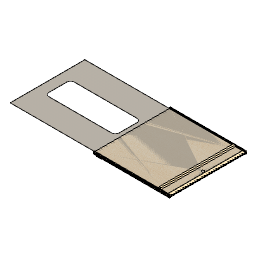
MKFG_DIYDoughLoader v2 (Autodesk Fusion 360 design; units mm, degrees)
Autodesk Fusion 360 part; units mm, degrees
sketch "Sketch1" plane through (0, 0, 0) normal (0, 1, 0) x (1, 0, 0) in component "ply_1/4_22x22"
  line L0 (-279.4, 279.4) -> (279.4, 279.4)
  line L1 (279.4, 279.4) -> (279.4, -279.4)
  line L2 (279.4, -279.4) -> (-279.4, -279.4)
  line L3 (-279.4, -279.4) -> (-279.4, 279.4)
  dimension "d1" = 558.8
  dimension "d2" = 558.8
  dimension "d3" = 279.4
  dimension "d4" = 279.4
  constraint horizontal L0
  constraint vertical L1
  constraint horizontal L2
  constraint vertical L3
  measures "d1" distance of L0.start L0.end
  measures "d2" distance of L0.start L2.end
  measures "d3" distance of origin L0
  measures "d4" distance of origin L3
extrude "Extrude1" add sketch "Sketch1" along normal blind 5.08 makes body 1 in component "ply_1/4_22x22"
sketch "Sketch1 (2)" plane through (0, 0, 0) normal (0, -1, 0) x (1, 0, 0) in component "Rails"
  line L0 (279.4, 279.4) -> (-279.4, 279.4)
  line L1 (-279.4, 279.4) -> (-279.4, -279.4)
  line L2 (-279.4, -279.4) -> (279.4, -279.4)
  line L3 (279.4, -279.4) -> (279.4, 279.4)
  line L4 (279.4, 273.05) -> (-279.4, 273.05)
  line L5 (-279.4, -273.05) -> (279.4, -273.05)
  dimension "d7" = -6.35
  dimension "d8" = -6.35
  constraint coincident L3 L5.end
  constraint perpendicular L3 L5
  constraint coincident L1 L5.start
  constraint coincident L3 L4.start
  constraint perpendicular L3 L4
  constraint coincident L1 L4.end
extrude "Extrude1'" add sketch "Sketch1 (2)" along normal blind 6.35 separate body contours L0 L1 L3 L4 | L1 L2 L3 L5 makes body 2 at (-93.1333, 0, -277.2833) makes body 3 at (-93.1333, 0, 275.1667) in component "Rails"
extrude "Extrude2" add sketch "Sketch1 (2)" against normal blind 6.35 from surface at -5.08 separate body contours L0 L1 L3 L4 | L1 L2 L3 L5 makes body 4 at (-93.1333, 5.08, -277.2833) makes body 5 at (-93.1333, 5.08, 275.1667) in component "Rails"
sketch "Sketch1 (3)" plane through (0, 0, -273.05) normal (0, 0, 1) x (1, 0, 0) in component "handle"
  line L0 (-279.4, 5.08) -> (279.4, 5.08)
  line L1 (279.4, 11.43) -> (-279.4, 11.43)
  line L2 (190.5, 5.08) -> (203.2, 5.08)
  line L3 (203.2, 5.08) -> (203.2, 17.78)
  line L4 (203.2, 17.78) -> (190.5, 17.78)
  line L5 (190.5, 17.78) -> (190.5, 5.08)
  line L6 (279.4, 5.08) -> (279.4, 11.43)
  line L7 (-279.4, 11.43) -> (-279.4, 5.08)
  dimension "d28" = 12.7
  dimension "d29" = 12.7
  dimension "d30" = 190.5
  constraint horizontal L2
  constraint vertical L3
  constraint horizontal L4
  constraint vertical L5
  constraint coincident L0 L2.start
  measures "d28" distance of L2.start L2.end
  measures "d29" distance of L2.start L4.end
  measures "d30" distance of origin L5
extrude "Extrude1''" add sketch "Sketch1 (3)" along normal blind 542.925 from surface at 1.5875 separate body contours L0 L1 L2 L3 L5 | L1 L3 L4 L5 makes body 6 in component "handle"
sketch "Sketch1 (4)" plane through (0, 5.08, 0) normal (0, 1, 0) x (-1, 0, 0) in component "Cloth"
  line L0 (279.4, 279.4) -> (-279.4, 279.4)
  line L1 (-279.4, -279.4) -> (279.4, -279.4)
  line L2 (-254, -271.4625) -> (279.4, -271.4625)
  line L3 (279.4, 271.4625) -> (-254, 271.4625)
  line L4 (-254, 271.4625) -> (-254, -271.4625)
  line L5 (279.4, -271.4625) -> (889, -271.4625)
  line L6 (304.8, -91.4625) -> (889, -91.4625)
  line L7 (889, -91.4625) -> (889, -271.4625)
  line L8 (889, -181.4625) -> (812.8, -181.4625) construction
  line L9 (889, -179.9625) -> (812.8, -179.9625)
  line L10 (889, -182.9625) -> (812.8, -182.9625)
  line L11 (812.8, -182.9625) -> (812.8, -179.9625)
  line L12 (279.4, 0) -> (325, 0) construction
  line L13 (304.8, 91.4625) -> (889, 91.4625)
  line L14 (279.4, 271.4625) -> (889, 271.4625)
  line L15 (889, 91.4625) -> (889, 271.4625)
  line L16 (889, 179.9625) -> (812.8, 179.9625)
  line L17 (889, 182.9625) -> (812.8, 182.9625)
  line L18 (812.8, 182.9625) -> (812.8, 179.9625)
  line L19 (889, -91.4625) -> (889, 91.4625)
  line L20 (812.8, -91.4625) -> (812.8, 91.4625)
  line L21 (-279.4, 279.4) -> (-279.4, -279.4)
  line L22 (279.4, -279.4) -> (279.4, 279.4)
  line L23 (304.8, -91.4625) -> (304.8, 91.4625)
  dimension "d43" = -7.9375
  dimension "d44" = -7.9375
  dimension "d47" = 609.6
  dimension "d48" = -180
  dimension "d49" = 76.2
  dimension "d50" = 1.5
  dimension "d51" = -1.5
  dimension "d56" = 76.2
  dimension "d59" = 25.4
  dimension "d60" = 25.4
  constraint coincident L3 L4.start
  constraint coincident L2 L4.end
  constraint perpendicular L2 L4
  constraint vertical L7
  constraint midpoint L7 L8.start
  constraint perpendicular L7 L8
  constraint perpendicular L9 L11
  constraint coincident L8.end L11
  constraint coincident L7 L10.start
  constraint coincident L7 L9.start
  constraint symmetric L2.end L12 L3.start
  constraint symmetric L5.end L12 L14.end
  constraint symmetric L6.start L12 L13.start
  constraint symmetric L6.end L12 L13.end
  constraint symmetric L9.start L12 L16.start
  constraint symmetric L9.end L12 L16.end
  constraint symmetric L10.start L12 L17.start
  constraint symmetric L10.end L12 L17.end
  constraint coincident L6 L20.start
  constraint coincident L13 L20.end
  constraint perpendicular L13 L20
  constraint midpoint L12.start L22
  constraint perpendicular L12 L22
  constraint coincident L2.end L22
  measures "d47" distance of L2.end L5.end
  measures "d49" distance of L8.start L8.end
  measures "d56" distance of L19 L20
  measures "d59" distance of L4 L21
  measures "d60" distance of L22 L23
extrude "Extrude1'''" add sketch "Sketch1 (4)" along normal blind 1.5 separate body contours L2 L3 L4 L22 | L5 L6 L7 L9 L10 L11 L13 L14 L15 L16 L17 L18 L22 L23 | L15 L16 L17 L18 | L7 L9 L10 L11 | L6 L13 L19 L20 makes body 7 in component "Cloth"
fillet "Fillet1" radius 25 4 edges at (-812.8, 5.83, -91.4625) (-812.8, 5.83, 91.4625) (-304.8, 5.83, -91.4625) (-304.8, 5.83, 91.4625) on bodies 7 in component "Cloth"
sketch "Sketch1 (5)" plane through (0, 0, 0) normal (0, -1, 0) x (1, 0, 0) in component "Bumpers_1/8x1/2"
  line L0 (279.4, 279.4) -> (-279.4, 279.4)
  line L1 (-279.4, 279.4) -> (-279.4, -279.4)
  line L2 (-279.4, -279.4) -> (279.4, -279.4)
  line L3 (279.4, -279.4) -> (279.4, 279.4)
  line L4 (-266.7, 279.4) -> (-266.7, -279.4)
  line L5 (266.7, -279.4) -> (266.7, 279.4)
  line L6 (279.4, 273.05) -> (-279.4, 273.05)
  line L7 (-279.4, -273.05) -> (279.4, -273.05)
  dimension "d61" = -12.7
  dimension "d62" = -12.7
  dimension "d63" = -6.35
  dimension "d64" = -6.35
extrude "Extrude1''''" add sketch "Sketch1 (5)" along normal blind 3.175 separate body contours L3 L5 L6 L7 | L1 L4 L6 L7 makes body 8 at (-275.1667, 0, 91.0167) makes body 9 at (270.9333, 0, 91.0167) in component "Bumpers_1/8x1/2"
fillet "Fillet1'" radius 3.175 4 edges at (-279.4, -3.175, 0) (-266.7, -3.175, 0) (279.4, -3.175, 0) (266.7, -3.175, 0) on bodies 8 9 in component "Bumpers_1/8x1/2"
fillet "Fillet3" radius 3.175 2 edges at (279.4, 5.08, 0) (-279.4, 5.08, 0) on bodies 1 in component "ply_1/4_22x22"
fillet "Fillet3'" radius 3.175 8 edges at (279.4, -6.35, -276.225) (-279.4, -6.35, -276.225) (279.4, 11.43, -276.225) (-279.4, 11.43, -276.225) (-279.4, -6.35, 276.225) (279.4, -6.35, 276.225) (-279.4, 11.43, 276.225) (279.4, 11.43, 276.225) on bodies 2 3 4 5 in component "Rails"
sketch "Sketch2" plane through (0, 5.08, 0) normal (0, 1, 0) x (-1, 0, 0) in component "ply_1/4_22x22"
  line L0 (276.225, -279.4) -> (276.225, 279.4)
  line L1 (276.225, 279.4) -> (-276.225, 279.4)
  line L2 (-276.225, 279.4) -> (-276.225, -279.4)
  line L3 (-276.225, -279.4) -> (276.225, -279.4)
  line L4 (-276.225, 0) -> (-238.125, 0)
  circle A0 centre (-238.125, 0) radius 9.525
  dimension "d71" = 38.1
  dimension "d72" = 19.05
  constraint midpoint L2 L4.start
  constraint perpendicular L2 L4
  constraint coincident L4.end A0.centre
  measures "d71" distance of L4.start L4.end
  measures "d72" diameter of A0
extrude "Extrude2'" cut sketch "Sketch2" against normal up to surface (5.08 mm away) contours A0 bodies 1 in component "ply_1/4_22x22"
sketch "Sketch1 (6)" plane through (0, 0, 279.4) normal (0, 0, 1) x (1, 0, 0) in component "DeckRest"
  arc A0 (276.225, -6.35) -> (279.4, -3.175) centre (276.225, -3.175) ccw
  line L0 (279.4, -3.175) -> (279.4, 0)
  line L1 (279.4, 0) -> (-279.4, 0)
  line L2 (-279.4, 0) -> (-279.4, -3.175)
  arc A1 (-279.4, -3.175) -> (-276.225, -6.35) centre (-276.225, -3.175) ccw
  line L3 (-276.225, -6.35) -> (276.225, -6.35)
  line L4 (-254, -6.35) -> (-215.9, -6.35)
  line L5 (-215.9, -6.35) -> (-215.9, -9.525)
  line L6 (-215.9, -9.525) -> (-254, -9.525)
  line L7 (-254, -9.525) -> (-254, -6.35)
  dimension "d98" = 38.1
  dimension "d99" = 3.175
  dimension "d100" = 25.4
  constraint horizontal L4
  constraint vertical L5
  constraint horizontal L6
  constraint vertical L7
  constraint coincident L3 L4.start
  measures "d98" distance of L4.start L4.end
  measures "d99" distance of L4.start L6.end
  measures "d100" horizontal distance of L1.end L4.start
extrude "Extrude1'''''" add sketch "Sketch1 (6)" against normal up to surface (558.8 mm away) separate body contours L3 L4 L5 L6 L7 makes body 10 in component "DeckRest"
fillet "Fillet1''" radius 1.5875 4 edges at (-254, -9.525, 0) (-254, -6.35, 0) (-215.9, -9.525, 0) (-215.9, -6.35, 0) on bodies 10 in component "DeckRest"
component "ply_1/4_22x22" placed x (1, 0, 0) y (0, 1, 0) z (0, 0, 1) at (0, 0, 0)
component "Rails" placed x (1, 0, 0) y (0, 1, 0) z (0, 0, 1) at (0, 0, 0)
component "handle" placed x (1, 0, 0) y (0, 1, 0) z (0, 0, 1) at (0, 0, 0)
component "Cloth" placed x (1, 0, 0) y (0, 1, 0) z (0, 0, 1) at (0, 0, 0)
component "Bumpers_1/8x1/2" placed x (1, 0, 0) y (0, 1, 0) z (0, 0, 1) at (0, 0, 0)
component "DeckRest" placed x (1, 0, 0) y (0, 1, 0) z (0, 0, 1) at (0, 0, 0)
equation "d1 = 22\""
equation "d2 = 22\""
equation "d3 = d2 / 2"
equation "d4 = d1 / 2"
equation "d31 = 0.125 in / 2"
equation "d32 = 10.375 in + 11\""
equation "d43 = -0.25 in - 1\" / 16"
equation "d44 = -0.25 in - 1\" / 16"
equation "d49 = 3\""
equation "d56 = 3\""
equation "d59 = 1\""
equation "d60 = 1\""
equation "d61 = -1\" / 2"
equation "d62 = -1\" / 2"
equation "d71 = 1\" + 0.5 in"
equation "d100 = 1\""
equation "d104 = 0.125 in / 2"
